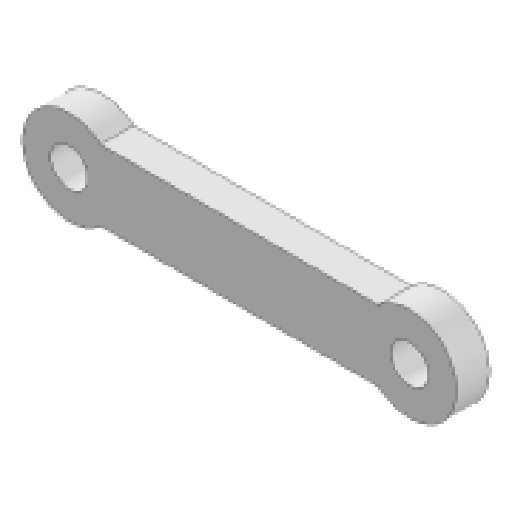
# Autodesk Inventor part: Arm 2
Saved by Autodesk Inventor 2025 (Build 290162010, 162A)
## iProperties
Created: 2024-11-29
Part Number: Arm 2
Material: Generic
Document SubType Name: Modeling
Designer: alexa
Density: 1 g/cm^3
Appearance: Default
Author: alexa
Autodesk Inventor part; units mm, degrees
ref_plane "YZ Plane" through (0, 0, 0) normal (1, 0, 0) x (0, 1, 0)
ref_plane "XZ Plane" through (0, 0, 0) normal (0, 1, 0) x (-1, 0, 0)
ref_plane "XY Plane" through (0, 0, 0) normal (0, 0, 1) x (1, 0, 0)
sketch "Sketch1" plane through (0, 0, 0) normal (0, 0, 1) x (1, 0, 0)
  arc A0 (3.3601, 3.81) -> (3.3601, -3.81) centre (0, 0) ccw
  line L0 (3.3601, 3.81) -> (33.3683, 3.81)
  line L1 (3.3601, -3.81) -> (33.3683, -3.81)
  arc A1 (33.3683, -3.81) -> (33.3683, 3.81) centre (36.7284, 0) ccw
  circle A2 centre (0, 0) radius 2.032
  circle A3 centre (36.7284, 0) radius 2.032
  dimension "d0" = 10.16
  dimension "d1" = 7.62
  dimension "d2" = 3.81
  dimension "d3" = 10.16
  dimension "d4" = 36.7284
  dimension "d5" = 4.064
  dimension "d6" = 4.064
  constraints: 4 centre point, 4 end point, 4 point on circle, 3 coincident, 2 horizontal, 1 horizontal alignment
  measures "d0" diameter of A0
  measures "d1" distance between parallel lines of L0 L1
  measures "d2" distance from line of point (0, 0) L1
  measures "d3" diameter of A1
  measures "d4" distance of A1.centre point (0, 0)
  measures "d5" diameter of A2
  measures "d6" diameter of A3
extrude "Extrusion1" add sketch "Sketch1" along normal blind 3.556
equation "\"d2\" = 0.5 * d1"
equation "\"d3\" = d0"
equation "\"d6\" = d5"
body "Solid1"
